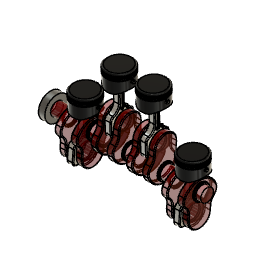
pistonsss v13 (Autodesk Fusion 360 design; units mm, degrees)
Autodesk Fusion 360 part; units mm, degrees
note: some values were not read from the file. Set by a fixed rule: which sketch regions a step uses; which face or edge a step refers to.
sketch "Sketch1" plane through (0, 0, 0) normal (0, 1, 0) x (1, 0, 0) in component "piston"
  line L0 (-20.4598, -70.312) -> (19.5402, -70.312)
  line L1 (19.5402, -70.312) -> (19.5402, -15.312)
  line L2 (19.5402, -15.312) -> (-20.4598, -15.312)
  line L3 (-20.4598, -15.312) -> (-20.4598, -70.312)
  line L4 (19.5402, -63.312) -> (15.5402, -63.312)
  line L5 (15.5402, -63.312) -> (15.5402, -61.312)
  line L6 (15.5402, -61.312) -> (19.5402, -61.312)
  line L7 (19.5402, -59.312) -> (15.5402, -59.312)
  line L8 (15.5402, -59.312) -> (15.5402, -57.312)
  line L9 (15.5402, -57.312) -> (19.5402, -57.312)
  line L10 (19.5402, -53.312) -> (15.5402, -53.312)
  line L11 (15.5402, -53.312) -> (15.5402, -51.312)
  line L12 (15.5402, -51.312) -> (19.5402, -51.312)
  dimension "d1" = 55
  dimension "d2" = 40
  dimension "d3" = 2
  dimension "d4" = 2
  dimension "d5" = 2
  dimension "d6" = 4
  dimension "d7" = 4
  dimension "d8" = 4
  dimension "d9" = 7
  dimension "d10" = 2
  dimension "d11" = 4
  constraint horizontal L0
  constraint vertical L1
  constraint horizontal L2
  constraint vertical L3
  constraint coincident L1 L4.start
  constraint perpendicular L1 L4
  constraint perpendicular L4 L5
  constraint coincident L1 L6.end
  constraint perpendicular L1 L6
  constraint coincident L1 L7.start
  constraint perpendicular L1 L7
  constraint perpendicular L7 L8
  constraint coincident L1 L9.end
  constraint perpendicular L1 L9
  constraint coincident L1 L10.start
  constraint perpendicular L1 L10
  constraint perpendicular L10 L11
  constraint coincident L1 L12.end
  constraint perpendicular L1 L12
  measures "d1" distance of L0.start L2.end
  measures "d2" distance of L0.start L0.end
  measures "d3" distance of L4.end L5.end
  measures "d4" distance of L7.end L8.end
  measures "d5" distance of L10.end L11.end
  measures "d6" distance of L4.start L4.end
  measures "d7" distance of L7.start L7.end
  measures "d8" distance of L10.start L10.end
  measures "d9" distance of L0 L4
  measures "d10" distance of L6 L7
  measures "d11" distance of L9 L10
revolve "Revolve1" add sketch "Sketch1" angle 360 about axis through (-20.4598, 0, 15.312) along (0, 0, 1) contours L0 L1 L2 L3 L4 L5 L6 L7 L8 L9 L10 L11 L12 makes body 1 in component "piston"
fillet "Fillet1" radius 5 1 edges at (-57.7529, -14.4646, 70.312) on bodies 1 in component "piston"
sketch "Sketch2" plane through (0, 0, 15.312) normal (0, 0, -1) x (1, 0, 0) in component "piston"
  circle A0 centre (-20.4598, 0) radius 40
  circle A1 centre (-20.4598, 0) radius 35
  dimension "d16" = 70
  constraint concentric A0 A1
  measures "d16" diameter of A1
extrude "Extrude1" cut sketch "Sketch2" against normal blind 50 contours A1 bodies 1 in component "piston"
sketch "Sketch3" plane through (0, 0, 0) normal (0, 1, 0) x (1, 0, 0) in component "piston"
  line L0 (-60.4598, -15.312) -> (19.5402, -15.312)
  line L1 (-60.4598, -51.312) -> (19.5402, -51.312)
  line L2 (-20.4598, -15.312) -> (-20.4598, -25.312)
  arc A0 (-55.9598, -15.312) -> (15.0402, -15.312) centre (-20.4598, 42.7005) ccw
  circle A1 centre (-20.4598, -39.312) radius 5
  dimension "d19" = 10
  dimension "d20" = 10
  dimension "d21" = 4.5
  dimension "d22" = 4.5
  dimension "d23" = 24
  constraint midpoint L0 L2.start
  constraint perpendicular L0 L2
  constraint coincident L2.end A0
  constraint coincident L0 A0.end
  constraint coincident L0 A0.start
  measures "d19" diameter of A1
  measures "d20" distance of L2.start L2.end
  measures "d21" distance of L0.start A0.start
  measures "d22" distance of L0.end A0.end
  measures "d23" distance of L2.start A1.centre
extrude "Extrude2" cut sketch "Sketch3" along normal mid plane 120 bodies 1 in component "piston"
pattern_linear "00000000-0000-0000-0000-000000000000" [suppressed] in component "pistons"
sketch "Sketch1 (2)" plane through (0, 0, 0) normal (1, 0, 0) x (0, 1, 0) in component "connectingrodsssss"
sketch "Sketch1 (3)" plane through (0, 0, 0) normal (1, 0, 0) x (0, 1, 0) in component "connectingrodss"
  circle A0 centre (49.5964, 67.6233) radius 5
  circle A1 centre (49.5964, 67.6233) radius 8.5
  circle A2 centre (49.5964, -57.3767) radius 22.5
  line L0 (49.5964, -57.3767) -> (13.5964, -57.3767)
  line L1 (13.5964, -57.3767) -> (13.5964, -32.3767)
  line L2 (41.1038, 67.9771) -> (41.1038, -7.33)
  line L3 (16.5331, -32.3263) -> (13.5964, -32.3767)
  arc A3 (16.5331, -32.3263) -> (41.1038, -7.33) centre (16.1038, -7.33) ccw
  line L4 (49.5964, 67.6233) -> (49.5964, -89.0874) construction
  line L5 (49.5964, -57.3767) -> (85.5964, -57.3767)
  line L6 (85.5964, -57.3767) -> (85.5964, -32.3767)
  line L7 (58.0964, 67.6233) -> (58.0964, -7.3767)
  line L8 (85.5964, -32.3767) -> (83.0964, -32.3767)
  arc A4 (58.0964, -7.3767) -> (83.0964, -32.3767) centre (83.0964, -7.3767) ccw
  line L9 (85.5964, -57.3767) -> (13.5964, -57.3767)
  line L10 (13.5964, -57.3767) -> (13.5964, -89.8767)
  line L11 (13.5964, -89.8767) -> (85.5964, -89.8767)
  line L12 (85.5964, -89.8767) -> (85.5964, -57.3767)
  circle A5 centre (49.5964, 52.6233) radius 4.75
  circle A6 centre (49.5964, -19.8767) radius 4.75
  line L13 (44.8464, 52.6233) -> (44.8464, -19.8767)
  line L14 (54.3464, 52.6233) -> (54.3464, -19.8767)
  dimension "d32" = 10
  dimension "d33" = 17
  dimension "d34" = 45
  dimension "d35" = 125
  dimension "d36" = 25
  dimension "d37" = 36
  dimension "d38" = 25
  dimension "d39" = 25
  dimension "d40" = 36
  dimension "d41" = 25
  dimension "d42" = 32.5
  dimension "d43" = 9.5
  dimension "d44" = 9.5
  dimension "d45" = 15
  dimension "d46" = 37.5
  constraint concentric A0 A1
  constraint coincident A2.centre L0.start
  constraint horizontal L0
  constraint perpendicular L0 L1
  constraint coincident A1 L2.start
  constraint vertical L2
  constraint tangent L2 A3
  constraint tangent L3 A3
  constraint coincident A0.centre A1.centre
  constraint perpendicular L0 L4
  constraint perpendicular L4 L5
  constraint perpendicular L5 L6
  constraint coincident A1 L7.start
  constraint tangent A1 L7
  constraint parallel L4 L7
  constraint horizontal L8
  constraint tangent L7 A4
  constraint tangent L8 A4
  constraint horizontal L9
  constraint vertical L10
  constraint horizontal L11
  constraint vertical L12
  constraint collinear L1 L10
  constraint coincident L4 A5.centre
  constraint coincident L4 A6.centre
  constraint coincident A5 L13.start
  constraint coincident A6 L13.end
  constraint tangent A6 L13
  constraint parallel L2 L13
  constraint coincident A5 L14.start
  constraint coincident A6 L14.end
  constraint tangent A6 L14
  constraint parallel L4 L14
  measures "d32" diameter of A0
  measures "d33" diameter of A1
  measures "d34" diameter of A2
  measures "d35" distance of A0.centre A2.centre
  measures "d36" distance of L0.end L1.end
  measures "d37" distance of A2.centre L0.end
  measures "d38" radius of A3
  measures "d39" distance of L5.end L6.end
  measures "d40" distance of A2.centre L5.end
  measures "d41" radius of A4
  measures "d42" distance of L5.end L11.end
  measures "d43" diameter of A5
  measures "d44" diameter of A6
  measures "d45" distance of A0.centre A5.centre
  measures "d46" distance of A2.centre A6.centre
extrude "Extrude1'" add sketch "Sketch1 (3)" along normal mid plane 20 separate body contours A1 L2 | A1 A2 L0 L1 L2 L3 A3 L5 L6 L7 L8 A4 L9 | A2 L0 L5 L9 L10 L11 L12 picked at (42.3347, 66.7239) makes body 2 in component "connectingrodss"
extrude "Extrude2'" add sketch "Sketch1 (3)" along normal mid plane 10 contours A5 | A5 A6 L13 L14 | A6 bodies 2 in component "connectingrodss"
fillet "Fillet1'" radius 12.5 4 edges at (0, 13.5964, -32.3767) (0, 13.5964, -89.8767) (0, 85.5964, -32.3767) (0, 85.5964, -89.8767) on bodies 2 in component "connectingrodss"
fillet "Fillet2" radius 2.5 12 edges at (-10, 58.0964, 30.1233) (-10, 63.2008, -22.515) (-10, 83.0442, -35.9497) (-10, 85.5964, -60.4478) (-10, 81.9352, -86.2156) (-10, 49.5964, -89.8767) (-10, 17.2576, -86.2156) (-10, 13.5964, -60.4254) (-10, 16.1494, -35.904) (-10, 35.9978, -22.4703) (-10, 41.1038, 30.3236) (-10, 49.7734, 76.1214) on bodies 2 in component "connectingrodss"
fillet "Fillet3" radius 2.5 12 edges at (10, 41.1038, 30.3236) (10, 35.9978, -22.4703) (10, 16.1494, -35.904) (10, 13.5964, -60.4254) (10, 17.2576, -86.2156) (10, 49.5964, -89.8767) (10, 81.9352, -86.2156) (10, 85.5964, -60.4478) (10, 83.0442, -35.9497) (10, 63.2008, -22.515) (10, 58.0964, 30.1233) (10, 49.7734, 76.1214) on bodies 2 in component "connectingrodss"
fillet "Fillet4" radius 1 4 edges at (-10, 49.5964, 57.3733) (-10, 44.8464, 16.3733) (-10, 49.5964, -24.6267) (-10, 54.3464, 16.3733) on bodies 2 in component "connectingrodss"
fillet "Fillet5" radius 1 4 edges at (10, 49.5964, 57.3733) (10, 54.3464, 16.3733) (10, 49.5964, -24.6267) (10, 44.8464, 16.3733) on bodies 2 in component "connectingrodss"
pattern_linear "00000000-0000-0000-0000-000000000000'" [suppressed] in component "connectingrodsssss"
sketch "Sketch1 (4)" plane through (0, 0, 0) normal (1, 0, 0) x (0, 1, 0) in component "pin"
cylinder "CylinderPrimitive1" add diameter 10 height 90 placed x (0, 0, -1) y (0, 1, 0) z (1, 0, 0) at (0, 32.1202, 105.1618) separate body makes body 3 in component "pin"
fillet "Fillet1''" radius 1.5 2 edges at (90, 30.3122, 109.8234) (0, 33.9283, 109.8234) on bodies 3 in component "pin"
pattern_linear "00000000-0000-0000-0000-000000000000''" [suppressed] in component "pinss"
sketch "Sketch1 (5)" plane through (0, 0, 0) normal (1, 0, 0) x (0, 1, 0) in component "crankshaft"
  circle A0 centre (30.6754, -101.5488) radius 22.5
  circle A1 centre (30.6754, -101.5488) radius 35
  circle A2 centre (28.5481, -37.0488) radius 20
  circle A3 centre (28.5481, -37.0488) radius 25
  arc A4 (83.5481, -59.0488) -> (-26.4519, -59.0488) centre (28.5481, -59.0488) ccw
  line L0 (65.6754, -101.5488) -> (65.6754, -59.0488)
  line L1 (-4.3246, -101.5488) -> (-4.3246, -59.0488)
  line L2 (-4.3246, -59.0488) -> (-26.4519, -59.0488)
  line L3 (65.6754, -59.0488) -> (83.5481, -59.0488)
  dimension "d73" = 70
  dimension "d75" = 42.5
  dimension "d76" = 40
  dimension "d77" = 50
  dimension "d78" = 22
  constraint concentric A0 A1
  constraint concentric A2 A3
  constraint coincident A1 L0.start
  constraint tangent A1 L0
  constraint coincident A1 L1.start
  constraint tangent A1 L1
  measures "d73" diameter of A1
  measures "d75" vertical distance of A0.centre A4.centre
  measures "d76" diameter of A2
  measures "d77" diameter of A3
  measures "d78" distance of A2.centre A4.centre
extrude "Extrude1''" add sketch "Sketch1 (5)" along normal blind 20 from surface at 15 separate body contours A0 | A1 | A1 A4 L0 L1 L2 L3 | A2 | A3 makes body 4 in component "crankshaft"
extrude "Extrude2''" add sketch "Sketch1 (5)" along normal blind 20 from surface at 35 contours A2 bodies 4 in component "crankshaft"
extrude "Extrude3" add sketch "Sketch1 (5)" along normal blind 5 from surface at 35 contours A3 bodies 4 in component "crankshaft"
fillet "Fillet1'''" radius 30 2 edges at (25, 65.6754, -59.0488) (25, -4.3246, -59.0488) on bodies 4 in component "crankshaft"
fillet "Fillet2'" radius 25 2 edges at (25, -26.4519, -59.0488) (25, 83.5481, -59.0488) on bodies 4 in component "crankshaft"
fillet "Fillet3'" radius 2.5 16 edges at (35, 65.6754, -94.0186) (35, 30.6754, -136.5488) (35, -4.3246, -94.7731) (35, -7.0744, -75.4505) (35, -23.0142, -51.4292) (35, 30.2999, -4.0767) (35, 80.9318, -52.8977) (35, 67.9058, -75.137) (15, -7.0744, -75.4505) (15, -4.3246, -94.7731) (15, 30.6754, -136.5488) (15, 65.6754, -94.0186) (15, 67.9058, -75.137) (15, 80.9318, -52.8977) (15, 30.2999, -4.0767) (15, -23.0142, -51.4292) on bodies 4 in component "crankshaft"
fillet "Fillet4'" radius 1.5 1 edges at (40, 5.2399, -46.0892) on bodies 4 in component "crankshaft"
mirror "Mirror1" about plane through (0, 0, 0) normal (1, 0, 0) of bodies 4 makes body 5 in component "crankshaft"
extrude "Extrude4" add sketch "Sketch1 (5)" along normal mid plane 40 contours A0 bodies 4 5 in component "crankshaft"
pattern_linear "R-Pattern1" count 4 spacing 110 along (-1, 0, 0) of bodies 4 makes body 6 at (-95, 3.5963, -54.9575) makes body 7 at (-205, 3.5963, -54.9575) makes body 8 at (-315, 3.5963, -54.9575) in component "crankshaft"
move_body "Move1" bodies 6 7 to x (1, 0, 0) y (0, -1, 0) z (0, 0, -1) at (0, 57.0962, -74.0976) in component "crankshaft"
combine "Combine1" operation add target body 7 tool bodies 8 4 6 in component "crankshaft"
extrude "Extrude5" add 1 faces at (-385, 30.7673, -41.8188) along direction (-1, 0, 0) blind 50 on bodies 7 bodies 7 in component "crankshaft"
sketch "Sketch1 (6)" plane through (-435, 0, 0) normal (-1, 0, 0) x (0, -1, 0)
  circle A0 centre (-28.5481, -37.0488) radius 20
  circle A1 centre (-28.5481, -37.0488) radius 37.5
  dimension "d106" = 75
  constraint concentric A0 A1
  measures "d106" diameter of A1
extrude "Extrude1'''" add sketch "Sketch1 (6)" against normal blind 20 separate body makes body 9 in component "Component"
sketch "Sketch1 (7)" plane through (0, 0, 0) normal (1, 0, 0) x (0, 1, 0) in component "piston (1)"
  line L0 (104.0463, 133.8476) -> (64.0463, 133.8476)
  line L1 (64.0463, 133.8476) -> (64.0463, 78.8476)
  line L2 (64.0463, 78.8476) -> (104.0463, 78.8476)
  line L3 (104.0463, 78.8476) -> (104.0463, 133.8476)
  line L4 (64.0463, 126.8476) -> (68.0463, 126.8476)
  line L5 (68.0463, 126.8476) -> (68.0463, 124.8476)
  line L6 (68.0463, 124.8476) -> (64.0463, 124.8476)
  line L7 (64.0463, 124.8476) -> (64.0463, 126.8476)
  line L8 (64.0463, 122.8476) -> (68.0463, 122.8476)
  line L9 (68.0463, 122.8476) -> (68.0463, 120.8476)
  line L10 (68.0463, 120.8476) -> (64.0463, 120.8476)
  line L11 (64.0463, 120.8476) -> (64.0463, 122.8476)
  line L12 (64.0463, 116.8476) -> (68.0463, 116.8476)
  line L13 (68.0463, 116.8476) -> (68.0463, 114.8476)
  line L14 (68.0463, 114.8476) -> (64.0463, 114.8476)
  line L15 (64.0463, 114.8476) -> (64.0463, 116.8476)
  dimension "d145" = 40
  dimension "d146" = 55
  dimension "d147" = 2
  dimension "d148" = 2
  dimension "d149" = 2
  dimension "d150" = 4
  dimension "d151" = 4
  dimension "d152" = 4
  dimension "d153" = 7
  dimension "d154" = 2
  dimension "d155" = 4
  constraint horizontal L0
  constraint vertical L1
  constraint horizontal L2
  constraint vertical L3
  constraint horizontal L4
  constraint vertical L5
  constraint horizontal L6
  constraint vertical L7
  constraint coincident L1 L4.start
  constraint horizontal L8
  constraint vertical L9
  constraint horizontal L10
  constraint vertical L11
  constraint coincident L1 L8.start
  constraint horizontal L12
  constraint vertical L13
  constraint horizontal L14
  constraint vertical L15
  constraint coincident L1 L12.start
  measures "d145" distance of L0.start L0.end
  measures "d146" distance of L0.start L2.end
  measures "d147" distance of L4.end L5.end
  measures "d148" distance of L8.end L9.end
  measures "d149" distance of L12.end L13.end
  measures "d150" distance of L5.end L6.end
  measures "d151" distance of L9.end L10.end
  measures "d152" distance of L13.end L14.end
  measures "d153" distance of L0 L4
  measures "d154" distance of L5.end L8
  measures "d155" distance of L10 L12
revolve "Revolve1'" add sketch "Sketch1 (7)" angle 360 about axis through (0, 104.0463, 78.8476) along (0, 0, 1) separate body contours L0 L1 L2 L3 L4 L5 L6 L8 L9 L10 L12 L13 L14 makes body 10 in component "piston (1)"
sketch "Sketch2 (2)" plane through (0, 0, 0) normal (1, 0, 0) x (0, 1, 0) in component "piston (1)"
sketch "Sketch3 (2)" plane through (0, 0, 78.8476) normal (0, 0, -1) x (1, 0, 0) in component "piston (1)"
  circle A0 centre (0, -104.0463) radius 40
  circle A1 centre (0, -104.0463) radius 35
  dimension "d158" = 70
  constraint concentric A0 A1
  measures "d158" diameter of A1
extrude "Extrude1''''" cut sketch "Sketch3 (2)" against normal blind 50 contours A1 bodies 10 in component "piston (1)"
fillet "Fillet1''''" radius 5 1 edges at (-37.2931, 89.5817, 133.8476) on bodies 10 in component "piston (1)"
sketch "Sketch4" plane through (0, 0, 0) normal (1, 0, 0) x (0, 1, 0) in component "piston (1)"
  line L0 (144.0463, 78.8476) -> (64.0463, 78.8476)
  line L1 (144.0463, 114.8476) -> (64.0463, 114.8476)
  line L2 (104.0463, 78.8476) -> (104.0463, 88.8476)
  arc A0 (139.5463, 78.8476) -> (68.5463, 78.8476) centre (104.0463, 20.8351) ccw
  circle A1 centre (104.0463, 106.1664) radius 5
  dimension "d163" = 10
  dimension "d164" = 4.5
  dimension "d165" = 4.5
  dimension "d166" = 10
  dimension "d167" = 17.3187
  dimension "d168" = 27.3187
  dimension "d169" = 17.3187
  dimension "d170" = 27.3187
  constraint midpoint L0 L2.start
  constraint perpendicular L0 L2
  constraint coincident L2.end A0
  constraint coincident L0 A0.start
  constraint coincident L0 A0.end
  measures "d163" distance of L2.start L2.end
  measures "d164" distance of L0.end A0.end
  measures "d165" distance of L0.start A0.start
  measures "d166" diameter of A1
  measures "d167" distance of L2.end A1.centre
  measures "d168" distance of L2.start A1.centre
  measures "d169" distance of L2.end A1.centre
  measures "d170" distance of L0 A1.centre
extrude "Extrude2'''" cut sketch "Sketch4" along normal mid plane 150 bodies 10 in component "piston (1)"
pattern_linear "00000000-0000-0000-0000-000000000000'''" [suppressed] in component "pistonsss"
sketch "Sketch2 (3)" plane through (0, -7.0979, 178.6796) normal (0, -0.039693, 0.999212) x (1, 0, 0)
  circle A0 centre (0.0024, 36.183) radius 35
  line L0 (-462.0011, 113.1658) -> (110.9697, 113.1658)
  line L1 (110.9697, 113.1658) -> (110.9697, -66.5233)
  line L2 (110.9697, -66.5233) -> (-462.0011, -66.5233)
  line L3 (-462.0011, -66.5233) -> (-462.0011, 113.1658)
  ellipse E0 centre (-334.9976, 37.5296) end of major axis (-374.9976, 37.5296) minor radius 39.9294
  ellipse E1 centre (-221.4976, 34.8723) end of major axis (-261.4976, 34.8723) minor radius 39.8279
  ellipse E2 centre (-114.9976, 34.8262) end of major axis (-74.9976, 34.8262) minor radius 39.802
  circle A1 centre (0.0024, 36.183) radius 40
  circle A2 centre (0.0024, 36.183) radius 47.5
  circle A3 centre (-114.9976, 34.8262) radius 47.5
  circle A4 centre (-221.4976, 34.8723) radius 47.5
  circle A5 centre (-334.9976, 37.5296) radius 47.5
  dimension "d203" = 95
  dimension "d204" = 95
  dimension "d205" = 95
  dimension "d206" = 95
  constraint horizontal L0
  constraint vertical L1
  constraint horizontal L2
  constraint vertical L3
  constraint concentric A1 A2
  constraint concentric E2 A3
  constraint concentric E1 A4
  constraint concentric E0 A5
  measures "d203" diameter of A2
  measures "d204" diameter of A3
  measures "d205" diameter of A4
  measures "d206" diameter of A5
extrude "Extrude1'''''" add sketch "Sketch2 (3)" along normal blind 25 separate body contours L0 L1 L2 L3 makes body 11 in component "Component'"
component "pistons" placed x (1, 0, 0) y (0, 1, 0) z (0, 0, 1) at (0, 0, 0)
component "connectingrodsssss" placed x (1, 0, 0) y (0, 1, 0) z (0, 0, 1) at (0, 0, 0)
component "pinss" placed x (1, 0, 0) y (0, 1, 0) z (0, 0, 1) at (0, 0, 0)
component "crankshaft" placed x (1, 0, 0) y (0, 0.99714, -0.075574) z (0, 0.075574, 0.99714) at (-5, 2.8816, 2.0515)
component "Component" placed x (1, 0, 0) y (0, 1, 0) z (0, 0, 1) at (0, 0, 0)
component "pistonsss" placed x (1, 0, 0) y (0, 1, 0) z (0, 0, 1) at (0, 0, 0)
component "Component'" placed x (1, 0, 0) y (0, 1, 0) z (0, 0, 1) at (0, 0, 0)
component "piston" placed x (1, 0, 0) y (0, 1, 0) z (0, 0, 1) at (211.252, 101.2847, -59.9792) in component "pistons"
component "piston" placed x (1, 0, 0) y (0, 1, 0) z (0, 0, 1) at (344.1119, 198.4777, -256.753) in component "pistons"
component "piston" placed x (1, 0, 0) y (0, 1, 0) z (0, 0, 1) at (422.1242, 159.8752, -205.5239) in component "pistons"
component "piston" placed x (1, 0, 0) y (0, 1, 0) z (0, 0, 1) at (448.8026, 112.8888, -163.1013) in component "pistons"
component "connectingrodss" placed x (1, 0, 0) y (0, 0.9998, 0.020015) z (0, -0.020015, 0.9998) at (-115, -19.4334, 83.8001) in component "connectingrodsssss"
component "connectingrodss" placed x (1, 0, 0) y (0, 0.997109, -0.075988) z (0, 0.075988, 0.997109) at (-5, -19.2982, -40.5455) in component "connectingrodsssss"
component "connectingrodss" placed x (1, 0, 0) y (0, 0.999807, 0.019646) z (0, -0.019646, 0.999807) at (-225, -19.4126, 83.8188) in component "connectingrodsssss"
component "connectingrodss" placed x (1, 0, 0) y (0, 0.996225, -0.086805) z (0, 0.086805, 0.996225) at (-335, -18.6338, -40.0597) in component "connectingrodsssss"
component "pin" placed x (1, 0, 0) y (0, -0.149979, 0.988689) z (0, -0.988689, -0.149979) at (-266.5, 137.6353, 136.4185) in component "pinss"
component "pin" placed x (1, 0, 0) y (0, 0.968251, 0.249982) z (0, -0.249982, 0.968251) at (-380, 31.8335, -86.8493) in component "pinss"
component "pin" placed x (1, 0, 0) y (0, 0.975438, -0.220275) z (0, 0.220275, 0.975438) at (-46.5, -19.2025, -72.39) in component "pinss"
component "pin" placed x (1, 0, 0) y (0, 0.761253, -0.648455) z (0, 0.648455, 0.761253) at (-160, -63.8446, 93.1763) in component "pinss"
component "piston (1)" placed x (1, 0, 0) y (0, 0.999212, 0.039693) z (0, -0.039693, 0.999212) at (-114.9976, -70.9507, 42.1899) in component "pistonsss"
component "piston (1)" placed x (1, 0, 0) y (0, 0.999212, 0.039693) z (0, -0.039693, 0.999212) at (-221.4976, -70.9046, 42.1908) in component "pistonsss"
component "piston (1)" placed x (1, 0, 0) y (0, 0.999212, 0.039693) z (0, -0.039693, 0.999212) at (-334.9976, -63.1049, -87.2095) in component "pistonsss"
component "piston (1)" placed x (1, 0, 0) y (0, 0.999212, 0.039693) z (0, -0.039693, 0.999212) at (0.0024, -64.457, -87.0991) in component "pistonsss"
